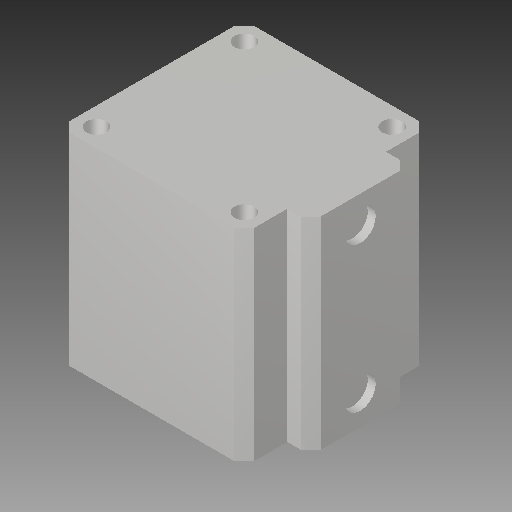
# Autodesk Inventor part: SDA 63 50
Saved by Autodesk Inventor 2019.4 (Build 234330000, 330)
## iProperties
Created: 2019-10-24
Part Number: SDA 63 50
Material: Aluminum 6061
Document SubType Name: Modeling
Designer: Mark
Density: 2.7 g/cm^3
Appearance: Aluminum - Flat
Author: Mark
Autodesk Inventor part; units mm, degrees
ref_plane "YZ Plane" through (0, 0, 0) normal (1, 0, 0) x (0, 1, 0)
ref_plane "XZ Plane" through (0, 0, 0) normal (0, 1, 0) x (-1, 0, 0)
ref_plane "XY Plane" through (0, 0, 0) normal (0, 0, 1) x (1, 0, 0)
sketch "Sketch1" plane through (0, 0, 0) normal (0, 1, 0) x (-1, 0, 0)
  line L0 (0, 0) -> (75, 0)
  line L1 (75, 0) -> (75, -75)
  line L2 (75, -75) -> (0, -75)
  line L3 (0, -75) -> (0, 0)
  dimension "d0" = 75
  dimension "d1" = 75
  constraints: 8 end point, 2 parallel, 1 horizontal, 1 perpendicular
  measures "d0" distance of L1.end L2.end
  measures "d1" distance of L0.end L1.end
extrude "Extrusion1" add sketch "Sketch1" along normal blind 82
sketch "Sketch2" plane through (0, 0, 0) normal (0, -1, 0) x (1, 0, 0)
  circle A0 centre (-37.5, -37.5) radius 20
  line L0 (0, -75) -> (0, 0) projected
  line L1 (-75, -75) -> (0, -75) projected
  dimension "d4" = 40
  dimension "d5" = 37.5
  dimension "d6" = 37.5
  constraints: 1 centre point
  measures "d4" diameter of A0
  measures "d5" distance from line of L0 A0.centre
  measures "d6" distance from line of L1 A0.centre
extrude "Extrusion2" add sketch "Sketch2" along normal blind 4
sketch "Sketch4" plane through (0, 0, 0) normal (0, -1, 0) x (1, 0, 0)
  circle A0 centre (-67.5, -7.5) radius 4
  circle A1 centre (-7.5, -7.5) radius 4
  circle A2 centre (-7.5, -67.5) radius 4
  circle A3 centre (-67.5, -67.5) radius 4
  line L0 (0, 0) -> (-75, 0) projected
  line L1 (0, -75) -> (0, 0) projected
  dimension "d12" = 8
  dimension "d13" = 8
  dimension "d14" = 8
  dimension "d15" = 8
  dimension "d16" = 60
  dimension "d17" = 60
  dimension "d18" = 60
  dimension "d19" = 60
  dimension "d20" = 60
  dimension "d21" = 60
  dimension "d22" = 7.5
  dimension "d23" = 7.5
  constraints: 4 centre point
  measures "d12" diameter of A0
  measures "d13" diameter of A1
  measures "d14" diameter of A2
  measures "d15" diameter of A3
  measures "d16" distance of A2.centre A3.centre
  measures "d17" distance of A1.centre A2.centre
  measures "d18" distance of A0.centre A1.centre
  measures "d19" distance of A3.centre A0.centre
  measures "d20" horizontal distance of A3.centre A1.centre
  measures "d21" horizontal distance of A2.centre A0.centre
  measures "d22" distance from line of L0 A1.centre
  measures "d23" distance from line of L1 A2.centre
extrude "Extrusion4" cut sketch "Sketch4" against normal blind 120.8875
sketch "Sketch5" plane through (0, 0, 0) normal (1, 0, 0) x (0, 0, -1)
  line L0 (75, 0) -> (0, 0) projected
  line L1 (75, 82) -> (0, 82) projected
  line L2 (17.5, 0) -> (57.5, 0)
  line L3 (57.5, 0) -> (57.5, 82)
  line L4 (57.5, 82) -> (17.5, 82)
  line L5 (17.5, 82) -> (17.5, 0)
  line L6 (0, 0) -> (0, 82) projected
  dimension "d26" = 40
  dimension "d27" = 17.5
  constraints: 8 end point, 2 parallel, 2 point on line, 1 horizontal, 1 perpendicular
  measures "d26" distance between parallel lines of L5 L3
  measures "d27" distance between parallel lines of L6 L5
extrude "Extrusion5" add sketch "Sketch5" along normal blind 9.5 contours L0 L5 L1 L3
sketch "Sketch6" plane through (9.5, 0, 0) normal (1, 0, 0) x (0, 0, -1)
  circle A0 centre (37.5, 12) radius 6.35
  circle A1 centre (37.5, 71) radius 6.35
  line L0 (57.5, 82) -> (17.5, 82) projected
  line L1 (75, 0) -> (57.5, 0) projected
  line L2 (75, 82) -> (0, 82) projected
  line L3 (37.5, 82) -> (37.5, 0)
  line L4 (0, 0) -> (75, 0) projected
  dimension "d30" = 12.7
  dimension "d31" = 12.7
  dimension "d32" = 11
  dimension "d33" = 12
  constraints: 2 centre point, 2 end point, 2 midpoint, 2 point on line
  measures "d30" diameter of A0
  measures "d31" diameter of A1
  measures "d32" distance from line of L0 A1.centre
  measures "d33" distance from line of L1 A0.centre
extrude "Extrusion6" cut sketch "Sketch6" against normal blind 3.2
chamfer "Chamfer1" distance 4 angle 45 4 edges at (0, 41, -75) (-75, 41, -75) (0, 41, 0) (-75, 41, 0)
chamfer "Chamfer2" distance 4 angle 45 2 edges at (9.5, 41, -17.5) (9.5, 41, -57.5)
body "Solid1"
